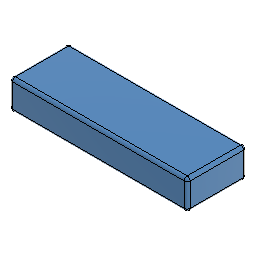
07-LargeWithLinkedComponents (Autodesk Fusion 360 archive; units mm, degrees)
design "07-LargeWithLinkedComponents_Source_01"
Autodesk Fusion 360 part; units mm, degrees
sketch "Sketch1" plane through (0, 0, 0) normal (0, 0, 1) x (1, 0, 0)
  line L0 (-30, 10) -> (30, 10)
  line L1 (30, 10) -> (30, 30)
  line L2 (30, 30) -> (-30, 30)
  line L3 (-30, 30) -> (-30, 10)
  line L4 (-30, 10) -> (30, 30) construction
  line L5 (30, 10) -> (-30, 30) construction
  point P0 (30, 10)
  point P1 (0, 20)
  dimension "d14" = 20
  dimension "d15" = 60
  constraint horizontal L0
  constraint perpendicular L0 L1
  constraint parallel L0 L2
  constraint parallel L1 L3
  constraint coincident L4 P1
  constraint coincident L5 P1
  constraint coincident P0 L0.end
  measures "d14" distance of P0 L1.end
  measures "d15" distance of L1.end L2.end
extrude "Extrude1" add sketch "Sketch1" along normal blind 10
fillet "Fillet1" radius 1 4 faces at (-10, 10, 3.3333) (-10, 23.3333, 10) (10, 30, 3.3333) (-10, 23.3333, 0)
